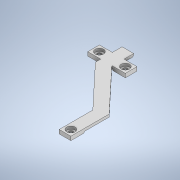
# Autodesk Inventor part: Cover_bottom_raceway_cover
Saved by Autodesk Inventor 2022 (Build 260153000, 153)
## iProperties
Created: 2021-08-04
Part Number: Cover_bottom_raceway_cover
Material: Generic
Document SubType Name: Modeling
Designer: exllu
Density: 1 g/cm^3
Appearance: Default
Author: exllu
Autodesk Inventor part; units mm, degrees
ref_plane "YZ Plane" through (0, 0, 0) normal (1, 0, 0) x (0, 1, 0)
ref_plane "XZ Plane" through (0, 0, 0) normal (0, 1, 0) x (-1, 0, 0)
ref_plane "XY Plane" through (0, 0, 0) normal (0, 0, 1) x (1, 0, 0)
sketch "Sketch1" plane through (0, 0, 0) normal (0, 1, 0) x (-1, 0, 0)
  line L0 (0, 0) -> (-10, 0)
  line L1 (-10, 0) -> (-10, -51)
  line L2 (-10, -51) -> (0, -51)
  line L3 (0, -51) -> (0, 0)
  line L4 (0, 0) -> (-41, 0)
  line L5 (-41, 0) -> (-41, -10)
  line L6 (-41, -10) -> (0, -10)
  line L7 (0, -10) -> (0, 0)
  line L8 (-41, -10) -> (-31, -10)
  line L9 (-31, -10) -> (-31, 30)
  line L10 (-31, 30) -> (-41, 30)
  line L11 (-41, 30) -> (-41, -10)
  line L12 (-10, -51) -> (-10, -43)
  line L13 (-10, -43) -> (-20, -43)
  line L14 (-20, -43) -> (10, -43)
  line L15 (10, -43) -> (10, -33)
  line L16 (10, -33) -> (-20, -33)
  line L17 (-20, -33) -> (-20, -43)
  point P0 (0, -43)
  point P1 (0, -33)
  point P2 (-31, 0)
  point P3 (-10, -10)
  point P4 (-10, -33)
  dimension "d0" = 10
  dimension "d1" = 51
  dimension "d2" = 41
  dimension "d3" = 10
  dimension "d4" = 10
  dimension "d5" = 40
  dimension "d6" = 8
  dimension "d7" = 10
  dimension "d8" = 30
  dimension "d9" = 10
  constraints: 36 end point, 8 parallel, 5 perpendicular, 4 horizontal, 1 point on line
  measures "d0" distance of L2.end L1.end
  measures "d1" distance of L1.end L0.end
  measures "d2" distance of L6.end L5.end
  measures "d3" distance of L5.end L4.end
  measures "d4" distance of L10.end L9.end
  measures "d5" distance of L9.end L8.end
  measures "d6" distance of L1.end L12.end
  measures "d7" distance of L12.end L13.end
  measures "d8" distance of L16.end L15.end
  measures "d9" distance of L15.end L14.end
extrude "Extrusion1" add sketch "Sketch1" along normal blind 3
sketch "Sketch2" plane through (0, 3, 0) normal (0, 1, 0) x (1, 0, 0)
  line L0 (-10, 33) -> (0, 33) projected
  line L1 (0, 33) -> (0, 38)
  line L2 (0, 38) -> (-5, 38)
  circle A0 centre (-5, 38) radius 3.25
  line L3 (0, 38) -> (15, 38)
  circle A1 centre (15, 38) radius 3.25
  line L4 (41, -30) -> (41, 10) projected
  line L5 (41, -30) -> (41, -25)
  line L6 (41, -25) -> (41, -30)
  line L7 (41, -25) -> (36, -25)
  circle A2 centre (36, -25) radius 3.25
  circle A3 centre (-5, 38) radius 1.7
  circle A4 centre (15, 38) radius 1.7
  circle A5 centre (36, -25) radius 1.7
  point P0 (0, 0)
  dimension "d12" = 5
  dimension "d13" = 5
  dimension "d14" = 6.5
  dimension "d15" = 15
  dimension "d16" = 6.5
  dimension "d17" = 5
  dimension "d18" = 5
  dimension "d19" = 5
  dimension "d20" = 6.5
  dimension "d23" = 3.4
  dimension "d24" = 3.4
  dimension "d25" = 3.4
  constraints: 12 end point, 6 centre point, 6 coincident, 2 horizontal, 1 collinear, 1 perpendicular, 1 point on line, 1 vertical
  measures "d12" distance of L0.end L1.end
  measures "d13" distance of L1.end L2.end
  measures "d14" diameter of A0
  measures "d15" distance of L1.end L3.end
  measures "d16" diameter of A1
  measures "d17" distance of L4.start L5.end
  measures "d18" distance of L5.end L4.start
  measures "d19" distance of L5.end L7.end
  measures "d20" diameter of A2
  measures "d23" diameter of A3
  measures "d24" diameter of A4
  measures "d25" diameter of A5
extrude "Extrusion3" cut sketch "Sketch2" against normal blind 2
extrude "Extrusion4" cut sketch "Sketch2" against normal blind 4 contours A3 | A4 | A5
sketch "Sketch3" plane through (0, 3, 0) normal (0, 1, 0) x (1, 0, 0)
  line L0 (0, 0) -> (0, 0.5)
  line L1 (0, 33) -> (0, 0) projected
  line L2 (0, 0.5) -> (31, 0.5)
  line L3 (31, 0.5) -> (31.5, 0.5)
  line L4 (31.5, 0.5) -> (31.5, -21.5)
  line L5 (31.5, -21.5) -> (40.5, -21.5)
  line L6 (31, -30) -> (41, -30) projected
  line L7 (40.5, -21.5) -> (40.5, 9.5)
  line L8 (41, -30) -> (41, 10) projected
  line L9 (40.5, 9.5) -> (9.5, 9.5)
  line L10 (9.5, 9.5) -> (9.5, 33.5)
  line L11 (9.5, 33.5) -> (19.5, 33.5)
  line L12 (20, 33) -> (20, 43) projected
  line L13 (19.5, 33.5) -> (19.5, 42.5)
  line L14 (19.5, 42.5) -> (9.5, 42.5)
  line L15 (9.5, 42.5) -> (9.5, 51)
  line L16 (10, 51) -> (0, 51) projected
  line L17 (10, 43) -> (10, 51) projected
  line L18 (9.5, 51) -> (10, 51)
  line L19 (10, 51) -> (10, 43)
  line L20 (20, 43) -> (10, 43) projected
  line L21 (20, 43) -> (10, 43)
  line L22 (10, 33) -> (20, 33) projected
  line L23 (20, 43) -> (20, 33)
  line L24 (20, 33) -> (10, 33)
  line L25 (10, 33) -> (10, 10)
  line L26 (41, 10) -> (10, 10) projected
  line L27 (10, 10) -> (41, 10)
  line L28 (41, 10) -> (41, -30)
  line L29 (31, 0) -> (31, -30) projected
  line L30 (41, -30) -> (31, -30)
  line L31 (31, -30) -> (31, 0)
  line L32 (31, 0) -> (0, 0)
  line L33 (0, 0.5) -> (0.5, 0.5)
  line L34 (0.5, 0.5) -> (0.5, 33.5)
  line L35 (9.5, 11.7035) -> (0.5, 11.7035)
  line L36 (5, 11.7035) -> (5, 17)
  line L37 (0.5, 9.5) -> (0.5, 33.5)
  line L38 (0.5, 33.5) -> (-9.5, 33.5)
  line L39 (-10, 33) -> (-10, 43)
  line L40 (-9.5, 33.5) -> (-9.5, 42.5)
  line L41 (-9.5, 42.5) -> (0.5, 42.5)
  line L42 (0.5, 42.5) -> (0.5, 51)
  line L43 (0, 51) -> (10, 51)
  line L44 (0, 43) -> (0, 51)
  line L45 (0.5, 51) -> (0, 51)
  line L46 (0, 51) -> (0, 43)
  line L47 (-10, 43) -> (0, 43)
  line L48 (-10, 43) -> (0, 43)
  line L49 (0, 33) -> (-10, 33)
  line L50 (-10, 43) -> (-10, 33)
  line L51 (-10, 33) -> (0, 33)
  line L52 (0, 33) -> (0, 10)
  line L53 (0, 0) -> (0.5, 0)
  line L54 (0.5, 0) -> (0.5, 33.5)
  line L55 (0.5, 33.5) -> (0, 33.5)
  line L56 (0, 33.5) -> (0, 0)
  dimension "d30" = 0.5
  dimension "d31" = 31
  dimension "d32" = 90
  dimension "d33" = 0.5
  dimension "d34" = 22
  dimension "d35" = 9
  dimension "d36" = 90
  dimension "d37" = 31
  dimension "d38" = 90
  dimension "d39" = 31
  dimension "d40" = 24
  dimension "d41" = 10
  dimension "d42" = 9
  dimension "d43" = 0.5
  constraints: 94 end point, 13 perpendicular, 11 point on line, 11 symmetric about line, 4 collinear, 4 parallel, 3 horizontal, 3 vertical, 1 midpoint
  measures "d30" distance of L0.start L0.end
  measures "d31" distance of L0.end L2.end
  measures "d32" angle of L0 L2
  measures "d33" distance of L2.end L3.end
  measures "d34" distance of L3.end L4.end
  measures "d35" distance of L4.end L5.end
  measures "d36" angle of L5 L4
  measures "d37" distance of L5.end L7.end
  measures "d38" angle of L7 L5
  measures "d39" distance of L7.end L9.end
  measures "d40" distance of L9.end L10.end
  measures "d41" distance of L10.end L11.end
  measures "d42" distance of L11.end L13.end
  measures "d43" distance of L0.end L33.end
extrude "Extrusion5" cut sketch "Sketch3" against normal blind 4 contours L0 L2 L54 L32 | L1 L56 L38 L34 L2 | L54 L2 L3 L4 L5 L7 L9 L10 L11 L13 L14 L15 L16 L17 L20 L12 L22 L25 L26 L8 L6 L29 L32 | L49 L39 L47 L44 L16 L42 L41 L40 L38 L56
sketch "Sketch4" plane through (0, 3, 0) normal (0, 1, 0) x (1, 0, 0)
  line L0 (40.5, 9.5) -> (40.5, 38.6053)
  line L1 (9.5, 33.5) -> (46.5578, 33.5)
  line L2 (40.5, 33.5) -> (40.5, 0.5)
  line L3 (40.5, 9.5) -> (40.5, -21.5) projected
  line L4 (9.5, 9.5) -> (9.5, 33.5) projected
  line L5 (40.5, 0) -> (9.5, 33)
  line L6 (40.5, 0) -> (33.9404, -6.1621)
  line L7 (33.9404, -6.1621) -> (-17.219, 48.2979)
  line L8 (0.5, 33.5) -> (0.5, 0.5) projected
  line L9 (0.5, 33) -> (0.5, 28.5562)
  line L10 (19.5, 33.5) -> (9.5, 33.5) projected
  line L11 (9.5, 33) -> (0.5, 33)
  line L12 (9.5, 33.5) -> (9.5, 33)
  line L13 (9.5, 33.5) -> (9.5, 9.5) projected
  point P0 (0, 0)
  point P1 (0.5, 29.4357)
  point P2 (0.5, 33)
  dimension "d49" = 33
  dimension "d50" = 9
  dimension "d55" = 0.5
  constraints: 18 end point, 3 point on line, 1 horizontal, 1 perpendicular, 1 vertical
  measures "d49" distance of L2.end L2.start
  measures "d50" distance of L5.start L6.end
  measures "d55" distance of L1.start L12.end
sketch "Sketch5" plane through (0, 3, 0) normal (0, 1, 0) x (1, 0, 0)
  line L0 (0.5, 33.5) -> (31.5, 33.5)
  line L1 (31.5, 33.5) -> (31.5, 9.5)
  line L2 (31.5, 0.5) -> (0.5, 0.5)
  line L3 (0.5, 0.5) -> (0.5, 33.5)
  line L4 (9.5, 9.5) -> (40.5, 9.5) projected
  line L5 (31.5, 0.5) -> (40.5, 0.5)
  line L6 (40.5, 0.5) -> (40.5, 9.5)
  line L7 (40.5, 9.5) -> (31.5, 9.5)
  point P0 (0, 0)
  constraints: 14 end point, 3 parallel, 2 horizontal, 2 perpendicular
extrude "Extrusion6" cut sketch "Sketch5" against normal blind 4
extrude "Extrusion7" add sketch "Sketch4" against normal blind 3 contours L6 L7 L4 L5 | L4 L7 L8 L11
sketch "Sketch6" plane through (0, 3, 0) normal (0, 1, 0) x (1, 0, 0)
  line L0 (40.0303, 0.5) -> (9.5, 33) projected
  line L1 (33.4215, 7.5352) -> (47.7617, -7.7302)
  line L2 (47.7617, -7.7302) -> (49.311, 2.3426)
  line L3 (49.311, 2.3426) -> (33.4215, 7.5352)
  line L4 (9.5, 33) -> (0.5, 33) projected
  line L5 (-9.5, 33.5) -> (19.5, 33.5) projected
  line L6 (0.5, 33) -> (9.5, 33)
  line L7 (9.5, 33) -> (9.5, 33.5)
  line L8 (9.5, 33.5) -> (0.5, 33.5)
  line L9 (0.5, 33.5) -> (0.5, 33)
  point P0 (0, 0)
  constraints: 14 end point, 2 parallel, 2 point on line, 1 collinear, 1 horizontal, 1 perpendicular
extrude "Extrusion8" add sketch "Sketch6" against normal blind 3 contours L4 L9 L5 L7
sketch "Sketch7" plane through (0, 3, 0) normal (0, 1, 0) x (1, 0, 0)
  line L0 (9.5, 33) -> (40.0303, 0.5) projected
  line L1 (37.6071, 3.0795) -> (42.3492, -1.9686)
  line L2 (42.3492, -1.9686) -> (43.0836, 1.6709)
  line L3 (43.0836, 1.6709) -> (37.6071, 3.0795)
  point P0 (0, 0)
  point P1 (40.0303, 0.5)
  constraints: 6 end point, 1 collinear, 1 point on line
extrude "Extrusion9" cut sketch "Sketch7" against normal blind 3
sketch "Sketch10" plane through (0, 3, 0) normal (0, 1, 0) x (1, 0, 0)
  line L0 (40.5, -21.5) -> (31.5, -21.5)
  line L1 (31.5, -21.5) -> (31.5, -29.5)
  line L2 (31.5, -29.5) -> (40.5, -29.5)
  line L3 (40.5, -29.5) -> (40.5, -21.5)
  point P0 (0, 0)
  dimension "d60" = 9
  dimension "d61" = 8
  constraints: 8 end point, 2 parallel, 1 horizontal, 1 perpendicular
  measures "d60" distance of L2.end L1.end
  measures "d61" distance of L1.end L0.end
extrude "Extrusion10" add sketch "Sketch10" against normal blind 3
sketch "Sketch11" plane through (0, 3, 0) normal (0, 1, 0) x (1, 0, 0)
  line L0 (31.5, -29.5) -> (40.5, -29.5) projected
  line L1 (36, -29.5) -> (36, -25)
  circle A0 centre (36, -25) radius 1.7
  point P0 (0, 0)
  dimension "d64" = 4.5
  dimension "d65" = 3.4
  constraints: 2 end point, 1 centre point, 1 coincident, 1 midpoint, 1 vertical
  measures "d64" distance of L1.start L1.end
  measures "d65" diameter of A0
extrude "Extrusion11" cut sketch "Sketch11" against normal blind 3
sketch "Sketch12" plane through (0, 3, 0) normal (0, 1, 0) x (1, 0, 0)
  circle A0 centre (36, -25) radius 1.7 projected
  circle A1 centre (36, -25) radius 3.25
  point P0 (0, 0)
  dimension "d68" = 6.5
  constraints: 1 centre point, 1 coincident
  measures "d68" diameter of A1
extrude "Extrusion12" cut sketch "Sketch12" against normal blind 2
sketch "Sketch13" plane through (0, 3, 0) normal (0, 1, 0) x (1, 0, 0)
  line L0 (9.5, 51) -> (9.5, 42.5) projected
  line L1 (0.5, 42.5) -> (0.5, 51) projected
  line L2 (9.5, 51) -> (0.5, 51)
  line L3 (0.5, 51) -> (0.5, 48.5)
  line L4 (0.5, 48.5) -> (9.5, 48.5)
  line L5 (9.5, 48.5) -> (9.5, 51)
  point P0 (0, 0)
  point P1 (9.5, 48.5)
  dimension "d71" = 2.5
  constraints: 8 end point, 2 parallel, 1 horizontal, 1 perpendicular, 1 point on line
  measures "d71" distance of L3.end L2.end
extrude "Extrusion13" cut sketch "Sketch13" against normal blind 3
sketch "Sketch14" plane through (0, 0, 0) normal (0, -1, 0) x (1, 0, 0)
  line L0 (9.5, -48.5) -> (0.5, -48.5) projected
  line L1 (9.5, -48.5) -> (0.5, -48.5)
  line L2 (0.5, -48.5) -> (0.5, -29.4357)
  line L3 (0.5, -29.4357) -> (9.5, -29.4357)
  line L4 (9.5, -29.4357) -> (9.5, -48.5)
  line L5 (-9.5, -33.5) -> (0.5, -33.5) projected
  line L6 (40.5, 29.5) -> (40.5, 0) projected
  line L7 (0.5, -33.5) -> (40.5, -33.5)
  line L8 (40.5, -33.5) -> (40.5, 19)
  line L9 (40.5, 19) -> (0.5, 19)
  line L10 (0.5, 19) -> (0.5, -33.5)
  point P0 (0, 0)
  point P1 (9.5, -33.5)
  point P2 (40.5, 0)
  dimension "d76" = 52.5
  constraints: 16 end point, 4 parallel, 2 horizontal, 2 perpendicular, 1 point on line
  measures "d76" distance of L8.end L7.end
extrude "Extrusion14" cut sketch "Sketch14" against normal blind 1
fillet "Fillet4" radius 1 3 edges at (0.5, 0, -38) (9.5, 0, -38) (36, 0, 19)
sketch "Sketch15" plane through (0, 1, 0) normal (0, -1, 0) x (1, 0, 0)
  line L0 (9.5, -42.5) -> (9.5, -48.5) projected
  line L1 (9.5, -48.5) -> (0.5, -48.5)
  line L2 (0.5, -48.5) -> (0.5, -50)
  line L3 (0.5, -50) -> (9.5, -50)
  line L4 (9.5, -50) -> (9.5, -48.5)
  point P0 (0, 0)
  dimension "d81" = 9
  dimension "d82" = 1.5
  constraints: 8 end point, 2 parallel, 1 horizontal, 1 perpendicular
  measures "d81" distance of L3.end L2.end
  measures "d82" distance of L2.end L1.end
extrude "Extrusion15" add sketch "Sketch15" against normal blind 2
fillet "Fillet6" radius 1.5 1 edges at (5, 1, -50)
body "Solid1"
